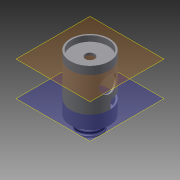
# Autodesk Inventor part: Mixture  Control
Saved by Autodesk Inventor 2015 (Build 190159000, 159)
## iProperties
Created: 2016-02-22
Part Number: Mixture  Control
Material: Generic
Document SubType Name: Modeling
Designer: 672301
Density: 1 g/cm^3
Appearance: Default
Author: 672301
Autodesk Inventor part; units mm, degrees
ref_plane "YZ Plane" through (0, 0, 0) normal (1, 0, 0) x (0, 1, 0)
ref_plane "XZ Plane" through (0, 0, 0) normal (0, 1, 0) x (-1, 0, 0)
ref_plane "XY Plane" through (0, 0, 0) normal (0, 0, 1) x (1, 0, 0)
sketch "Sketch1" plane through (0, 0, 0) normal (0, 1, 0) x (-1, 0, 0)
  circle A0 centre (0, 0) radius 5.2959
  dimension "d0" = 10.5918
  constraints: 1 centre point, 1 coincident
  measures "d0" diameter of A0
extrude "Extrusion1" add sketch "Sketch1" along normal blind 15.0368
sketch "Sketch3" plane through (0, 15.0368, 0) normal (0, 1, 0) x (1, 0, 0)
  circle A0 centre (0, 0) radius 3.4925
  dimension "d6" = 6.985
  constraints: 1 centre point, 1 coincident
  measures "d6" diameter of A0
extrude "Extrusion3" add sketch "Sketch3" against normal blind 15.2908
sketch "Sketch4" plane through (0, 15.0368, 0) normal (0, 1, 0) x (1, 0, 0)
  circle A0 centre (0, 0) radius 3.175
  dimension "d9" = 6.35
  constraints: 1 centre point, 1 coincident
  measures "d9" diameter of A0
extrude "Extrusion4" add sketch "Sketch4" against normal blind 18.7706
sketch "Sketch9" plane through (0, -3.7338, 0) normal (0, -1, 0) x (1, 0, 0)
  circle A0 centre (0, 0) radius 5.2959 projected
hole "Hole1" at (0, -3.7338, 0) direction (0, 1, 0) diameter 2.4892 end through all
sketch "Sketch10" plane through (0, 0, 0) normal (1, 0, 0) x (0, 1, 0)
  line L0 (15.0368, -5.2959) -> (15.0368, 5.2959) projected
  line L1 (15.0368, -5.256) -> (9.6521, -5.2959)
  line L2 (0, -5.2959) -> (15.0368, -5.2959) projected
  circle A0 centre (9.6521, 0) radius 2.286
  point P0 (0, 0)
  dimension "d33" = 5.3848
  dimension "d34" = 4.572
  constraints: 2 end point, 2 point on line, 1 centre point
  measures "d33" distance of L1.start L1.end
  measures "d34" diameter of A0
extrude "Extrusion7" cut sketch "Sketch10" along normal mid plane 12.446 contours A0
sketch "Sketch5" plane through (0, 15.0368, 0) normal (0, 1, 0) x (1, 0, 0)
  circle A0 centre (0, 0) radius 4.8768
  dimension "d12" = 9.7536
  constraints: 1 centre point, 1 coincident
  measures "d12" diameter of A0
extrude "Extrusion5" cut sketch "Sketch5" against normal blind 1.524
ref_plane "Work Plane3" through (0, 12.9032, 0) normal (0, 1, 0) x (-1, 0, 0)
sketch "Sketch8" plane through (0, 12.9032, 0) normal (0, 1, 0) x (-1, 0, 0)
  circle A0 centre (0, 0) radius 4.8768
  constraints: 1 centre point, 1 coincident
extrude "Extrusion6" cut sketch "Sketch8" against normal blind 12.446
ref_plane "Work Plane4" through (0, 3.6322, 0) normal (0, -1, 0) x (1, 0, 0)
chamfer "Chamfer1" distance 0.508 angle 45 1 edges at (-3.175, -3.7338, 0)
sketch "Sketch11" plane through (0, 3.6322, 0) normal (0, -1, 0) x (1, 0, 0)
  circle A0 centre (0, 0) radius 5.2959 projected
  circle A1 centre (0, 0) radius 4.8768 projected
  line L0 (4.8768, 0) -> (1.7044, -4.5693)
  line L1 (2.1158, -4.8549) -> (5.2959, -0.291)
  line L2 (4.8768, 0) -> (5.9401, -0.7399)
  line L3 (5.9401, -0.7399) -> (2.763, -5.3059)
  line L4 (2.763, -5.3059) -> (1.7044, -4.5693)
  dimension "d37" = 5.5626
  dimension "d38" = 1.2954
  constraints: 10 end point, 3 point on circle, 2 perpendicular, 2 other
  measures "d37" distance of L0.start L0.end
  measures "d38" distance of L0.start L2.end
extrude "Extrusion8" cut sketch "Sketch11" against normal blind 2.159 contours L1 A1 A0 | L4 A1 L1 | A0 L1 L2 L3 L4 | L2 L1 A0 | A0 L1 A1 L2 | L1 A1 | A1 L0 L1 | A1 L0
thread "Thread1" size "1/4-20 UNC" class "2A" standard "ANSI Unified Screw Threads" full length
body "Solid1"
